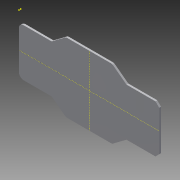
# Autodesk Inventor part: Basetrimed
Saved by Autodesk Inventor 2015 (Build 190159000, 159)
## iProperties
Created: 2014-11-04
Part Number: Basetrimed
Material: ABS Plastic
Document SubType Name: Modeling
Designer: ah14592
Density: 1.06 g/cm^3
Appearance: Smooth - White
Author: ah14592
Autodesk Inventor part; units mm, degrees
sketch "Sketch1" plane through (0, 0, 0) normal (0, 1, 0) x (-1, 0, 0)
  line L0 (0, 0) -> (-300, 0)
  line L1 (-300, 0) -> (-300, -148)
  line L2 (-300, -148) -> (0, -148)
  line L3 (0, -148) -> (0, 0)
  dimension "d0" = 300
  dimension "d1" = 148
  constraints: 8 end point, 2 parallel, 1 horizontal, 1 perpendicular
  measures "d0" distance of L2.end L1.end
  measures "d1" distance of L1.end L0.end
extrude "Extrusion1" add sketch "Sketch1" along normal blind 4
sketch "Sketch2" plane through (0, 0, 0) normal (0, -1, 0) x (1, 0, 0)
  line L0 (0, -74) -> (300, -74) construction
  line L1 (150, 0) -> (150, -148) construction
  constraints: 4 end point
sketch "Sketch3" plane through (0, 0, 0) normal (0, -1, 0) x (1, 0, 0)
  line L0 (0, -148) -> (70, -148)
  line L1 (70, -148) -> (70, -125)
  line L2 (70, -125) -> (0, -125)
  line L3 (0, -125) -> (0, -148)
  point P0 (0, 0)
  dimension "d4" = 70
  dimension "d5" = 23
  constraints: 8 end point, 2 parallel, 1 horizontal, 1 perpendicular
  measures "d4" distance of L2.end L1.end
  measures "d5" distance of L1.end L0.end
extrude "Extrusion2" cut sketch "Sketch3" against normal blind 10
fillet "Fillet1" radius 10 1 edges at (0, 2, -125)
sketch "Sketch4" plane through (0, 0, 0) normal (0, -1, 0) x (1, 0, 0)
  line L0 (70, -125) -> (100.659, -148)
  line L1 (300, -148) -> (70, -148) projected
  line L2 (70, -148) -> (70, -125)
  line L3 (70, -125) -> (70, -148) projected
  point P0 (0, 0)
  constraints: 4 end point, 1 collinear, 1 point on line
extrude "Extrusion3" cut sketch "Sketch4" against normal blind 10
ref_plane "Work Plane1" through (150, 0, 0) normal (1, 0, 0) x (0, 0, -1)
ref_plane "Work Plane2" through (100.659, 0, -74) normal (0, 0, -1) x (-1, 0, 0)
mirror "Mirror2" about plane through (100.659, 0, -74) normal (0, 0, -1) of "Extrusion2", "Extrusion3"
fillet "Fillet2" radius 10 1 edges at (0, 2, -23)
sketch "Sketch6" plane through (0, 0, 0) normal (0, -1, 0) x (1, 0, 0)
  point P0 (0, 0)
ref_plane "Work Plane3" through (150, 0, 0) normal (1, 0, 0) x (0, 0, -1)
mirror "Mirror3" about plane through (150, 0, 0) normal (1, 0, 0) of "Extrusion2", "Extrusion3", "Mirror2"
chamfer "Chamfer1" distance 8 angle 45 2 edges at (300, 2, -23) (300, 2, -125)
fillet "Fillet3" radius 8 4 edges at (199.341, 2, 0) (100.659, 2, 0) (199.341, 2, -148) (100.659, 2, -148)
sketch "Sketch7" plane through (0, 4, 0) normal (0, 1, 0) x (1, 0, 0)
  point P0 (0, 0)
body "Solid1"
